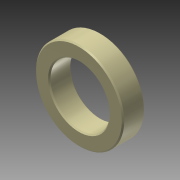
# Autodesk Inventor part: am-2271
Saved by Autodesk Inventor 2013 (Build 170138000, 138)
## iProperties
Category: Drive Base Kit
Company: Autodesk Inc.
Created: 2012-12-22
Part Number: am-2271
Document SubType Name: Modeling
Designer: Autodesk Inc.
Density: 1.10705 g/cm^3
Material: Nylon-6/6
Mass: 0.816466 g
Surface Area: 7.60009 cm^2
Volume: 0.737515 cm^3
Catalog Web Link: http://www.andymark.com/ProductDetails.asp?ProductCode=am-1181
Description: 0.188 inch thick spacer, 1/2" nominal id, made from Nylon
Vendor: AndyMark
Author: Autodesk Inc.
Autodesk Inventor part; units mm, degrees
ref_plane "YZ Plane" through (0, 0, 0) normal (1, 0, 0) x (0, 1, 0)
ref_plane "XZ Plane" through (0, 0, 0) normal (0, 1, 0) x (-1, 0, 0)
ref_plane "XY Plane" through (0, 0, 0) normal (0, 0, 1) x (1, 0, 0)
sketch "Sketch1" plane through (0, 0, 0) normal (0, 0, 1) x (1, 0, 0)
  circle A0 centre (0, 0) radius 6.4135
  circle A1 centre (0, 0) radius 9.525
  dimension "d0" = 12.827
  dimension "d1" = 19.05
  constraints: 2 centre point, 2 coincident
  measures "d0" diameter of A0
  measures "d1" diameter of A1
extrude "Extrusion1" add sketch "Sketch1" against normal blind 4.7752
chamfer "Chamfer1" distance 0.254 angle 45 4 edges at (-9.525, 0, 0) (-6.4135, 0, 0) (-9.525, 0, -4.7752) (-6.4135, 0, -4.7752)
body "Solid1"
